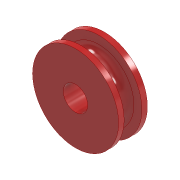
# Autodesk Inventor part: plastic pulley deep u
Saved by Autodesk Inventor 2020 (Build 240168000, 168)
## iProperties
Created: 2019-11-14
Part Number: plastic pulley deep u
Material: Generic
Document SubType Name: Modeling
Designer: ball
Density: 1 g/cm^3
Appearance: Default
Author: ball
Autodesk Inventor part; units mm, degrees
ref_plane "YZ Plane" through (0, 0, 0) normal (1, 0, 0) x (0, 1, 0)
ref_plane "XZ Plane" through (0, 0, 0) normal (0, 1, 0) x (-1, 0, 0)
sketch "Sketch1" plane through (0, 0, 0) normal (0, 1, 0) x (-1, 0, 0)
  line L0 (5.9801, -2.0066) -> (-0.0143, -2.0066)
  line L1 (5.9801, 2.0066) -> (-0.0143, 2.0066)
  line L2 (5.9801, 1.2446) -> (4.8625, 1.2446)
  line L3 (4.8625, 2.0066) -> (4.8625, -2.0066) construction
  line L4 (5.9801, 2.0066) -> (5.9801, 1.2446)
  line L5 (5.9801, -1.2446) -> (5.9801, -2.0066)
  line L6 (-0.0143, 2.0066) -> (-0.0143, -2.0066)
  line L7 (0, 0) -> (5.9944, 0) construction
  line L8 (3.6179, 2.0066) -> (3.6179, -2.0066) construction
  arc A0 (4.8625, 1.2446) -> (4.8625, -1.2446) centre (4.8625, 0) ccw
  line L9 (5.9801, -1.2446) -> (4.8625, -1.2446)
  line L10 (-0.0143, -1.2446) -> (-0.046, -1.2446)
  dimension "d4" = 0.762
  dimension "d6" = 2.0066
  dimension "d7" = 2.0066
  dimension "d9" = 1.1176
  dimension "d10" = 5.9944
  dimension "d11" = 5.9944
  dimension "d12" = 0.762
  dimension "d13" = 1.2446
  dimension "d15" = 1.2446
  constraints: 22 end point, 7 point on line, 2 perpendicular, 2 point on circle, 1 centre point, 1 horizontal, 1 vertical
  measures "d4" distance from line of L5.start L0
  measures "d6" distance from line of L0 L7.start
  measures "d7" distance from line of L1 L7.start
  measures "d9" distance between parallel lines of L3 L5
  measures "d10" distance between parallel lines of L6 L5
  measures "d11" distance between parallel lines of L6 L4
  measures "d12" distance between parallel lines of L2 L1
  measures "d13" distance between parallel lines of L7 L2
  measures "d15" distance between parallel lines of L8 L3
revolve "Revolution1" add sketch "Sketch1" angle 360 about axis through (0.0143, 0, 2.0066) along (0, 0, -1)
sketch "Sketch2" plane through (0.0143, 0, -2.0066) normal (0, 0, -1) x (-1, 0, 0)
  circle A0 centre (0.0143, 0) radius 1.7
  dimension "d17" = 3.4
  constraints: 1 centre point, 1 coincident
  measures "d17" diameter of A0
extrude "Extrusion1" cut sketch "Sketch2" against normal through all
ref_plane "Work Plane1" through (0.0143, 0, 0) normal (0, 0, 1) x (1, 0, 0)
equation "\"d7\" = d6"
equation "\"d11\" = d10"
equation "\"d12\" = d4"
equation "\"d15\" = d14"
equation "\"d14\" = 1.2446"
body "Solid1"
